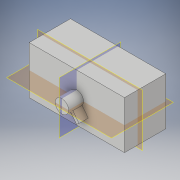
# Autodesk Inventor part: Assembly Mount Base
Saved by Autodesk Inventor 2019 (Build 230136000, 136)
## iProperties
Created: 2021-02-18
Part Number: Assembly Mount Base
Material: Generic
Document SubType Name: Modeling
Designer: Eric
Density: 1 g/cm^3
Appearance: Default
Author: Eric
Autodesk Inventor part; units mm, degrees
ref_plane "YZ Plane" through (0, 0, 0) normal (1, 0, 0) x (0, 1, 0)
ref_plane "XZ Plane" through (0, 0, 0) normal (0, 1, 0) x (-1, 0, 0)
ref_plane "XY Plane" through (0, 0, 0) normal (0, 0, 1) x (1, 0, 0)
sketch "Sketch1" plane through (0, 0, 0) normal (0, 0, 1) x (1, 0, 0)
  line L0 (0, 0) -> (300, 0)
  line L1 (300, 0) -> (300, -150)
  line L2 (300, -150) -> (0, -150)
  line L3 (0, -150) -> (0, 0)
  dimension "d0" = 300
  dimension "d1" = 150
  constraints: 8 end point, 3 perpendicular, 1 horizontal
  measures "d0" distance of L1.end L2.end
  measures "d1" distance of L0.end L1.end
extrude "Extrusion1" add sketch "Sketch1" along normal blind 130
sketch "Sketch2" plane through (0, 0, 130) normal (0, 0, 1) x (1, 0, 0)
  line L0 (0, -150) -> (300, -150) projected
  line L1 (0, 0) -> (300, -150) construction
  line L2 (0, -150) -> (300, 0) construction
  circle A0 centre (150, -75) radius 21
  line L3 (166.513, -87.9739) -> (186.0161, -112.874)
  line L4 (186.0161, -112.874) -> (178.1436, -119.0402)
  line L5 (178.1436, -119.0402) -> (158.6404, -94.1401)
  line L6 (158.6404, -94.1401) -> (166.513, -87.9739)
  line L7 (162.5767, -91.057) -> (182.0799, -115.9571) construction
  line L8 (150, -75) -> (205.4242, -145.7614) construction
  dimension "d4" = 42
  dimension "d5" = 52.025
  dimension "d6" = 51.93
  dimension "d7" = 10
  constraints: 16 end point, 3 midpoint, 3 perpendicular, 1 collinear, 3 other
  measures "d5" distance from line of L8.start L4
  measures "d6" angle of L0 L5
  measures "d7" distance between parallel lines of L3 L5
extrude "Extrusion2" add sketch "Sketch2" along normal blind 47 separate body contours A0 L6 | L6 A0
extrude "Extrusion3" add sketch "Sketch2" along normal blind 29 separate body contours L6 A0 | A0 L3 L4 L5 picked at (163.1281, -90.8523)
ref_plane "Work Plane1" through (150, -75, 88.5) normal (0, 0, 1) x (1, 0, 0)
ref_plane "Work Plane2" through (0, -75, 0) normal (0, 1, 0) x (1, 0, 0)
ref_plane "Work Plane3" through (150, -150, 0) normal (-1, 0, 0) x (0, 0, 1)
body "Solid1"
body "Solid2"
body "Solid3"
